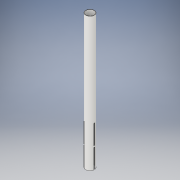
# Autodesk Inventor part: Body
Saved by Autodesk Inventor 2018 (Build 220112000, 112)
## iProperties
Created: 2017-10-02
Part Number: Body
Material: Generic
Document SubType Name: Modeling
Designer: Intel
Density: 1 g/cm^3
Appearance: White
Author: Intel
Autodesk Inventor part; units mm, degrees
ref_plane "YZ Plane" through (0, 0, 0) normal (1, 0, 0) x (0, 1, 0)
ref_plane "XZ Plane" through (0, 0, 0) normal (0, 1, 0) x (-1, 0, 0)
ref_plane "XY Plane" through (0, 0, 0) normal (0, 0, 1) x (1, 0, 0)
sketch "Sketch1" plane through (0, 0, 0) normal (0, 1, 0) x (-1, 0, 0)
  circle A0 centre (0, 0) radius 36.5125
  circle A1 centre (0, 0) radius 39.6875
  dimension "d0" = 73.025
  dimension "d1" = 79.375
  constraints: 2 centre point, 2 coincident
  measures "d0" diameter of A0
  measures "d1" diameter of A1
extrude "Extrusion1" add sketch "Sketch1" along normal mid plane 1219.2
sketch "Sketch2" plane through (0, 0, 0) normal (1, 0, 0) x (0, 1, 0)
  line L0 (-609.6, 4.7625) -> (-431.8, 4.7625)
  line L1 (-431.8, 4.7625) -> (-431.8, -4.7625)
  line L2 (-431.8, -4.7625) -> (-609.6, -4.7625)
  line L3 (-609.6, -4.7625) -> (-609.6, 4.7625)
  line L4 (-609.6, 39.6875) -> (-609.6, -39.6875) projected
  line L5 (-609.6, 39.6875) -> (-609.6, -39.6875) projected
  line L6 (609.6, -39.6875) -> (609.6, 39.6875) projected
  line L7 (-609.6, -39.6875) -> (609.6, -39.6875) projected
  line L8 (-419.1, 4.7625) -> (-241.3, 4.7625)
  line L9 (-241.3, 4.7625) -> (-241.3, -4.7625)
  line L10 (-241.3, -4.7625) -> (-419.1, -4.7625)
  line L11 (-419.1, -4.7625) -> (-419.1, 4.7625)
  point P0 (0, 0)
  dimension "d4" = 177.8
  dimension "d5" = 9.525
  dimension "d6" = 34.925
  dimension "d12" = 177.8
  dimension "d13" = 9.525
  dimension "d14" = 12.7
  constraints: 16 end point, 4 parallel, 2 collinear, 2 horizontal, 2 perpendicular
  measures "d4" distance of L1.end L2.end
  measures "d5" distance of L2.end L0.start
  measures "d6" distance between parallel lines of L7 L2
  measures "d12" distance of L9.end L10.end
  measures "d13" distance of L10.end L8.start
  measures "d14" distance between parallel lines of L1 L11
extrude "Extrusion2" cut sketch "Sketch2" along normal blind 76.2
pattern_circular "Circular Pattern1" count 3 over 360 about axis through (0, 0, 0) along (0, 1, 0) of "Extrusion2"
equation "\"d13\" = d5"
body "Solid1"
